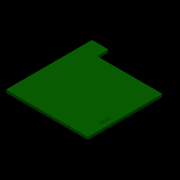
# Autodesk Inventor part: hw_DAA - PCB Power
Saved by Autodesk Inventor 2018 (Build 220112000, 112)
## iProperties
Created: 2024-03-13
Part Number: hw_DAA - PCB Power
Material: PCB
Document SubType Name: Modeling
Designer: cda1
Density: 4 g/cm^3
Appearance: PCB
Author: cda1
Autodesk Inventor part; units mm, degrees
ref_plane "YZ Plane" through (0, 0, 0) normal (1, 0, 0) x (0, 1, 0)
ref_plane "XZ Plane" through (0, 0, 0) normal (0, 1, 0) x (-1, 0, 0)
sketch "Boceto1" plane through (0, 0, 0) normal (0, 0, 1) x (1, 0, 0)
  line L0 (-26, 26) -> (26, 26)
  line L1 (26, 26) -> (26, -26)
  line L2 (26, -26) -> (-26, -26)
  line L3 (-26, -26) -> (-26, 26)
  line L4 (-26, 26) -> (26, -26) construction
  line L5 (26, 26) -> (-26, -26) construction
  point P0 (0, 0)
  dimension "d0" = 52
  dimension "d1" = 52
  constraints: 12 end point, 2 midpoint, 2 parallel, 1 horizontal, 1 perpendicular
  measures "d0" distance of L1.end L2.end
  measures "d1" distance of L0.end L1.end
extrude "Extrusión1" add sketch "Boceto1" against normal blind 1.742
fillet "Empalme1" radius 0.5 4 edges at (26, 26, -0.871) (-26, 26, -0.871) (-26, -26, -0.871) (26, -26, -0.871)
ref_plane "Plano de trabajo1" through (0, 0, -1.6) normal (0, 0, 1) x (1, 0, 0)
sketch "Boceto6" plane through (0, 0, 0) normal (0, 0, 1) x (1, 0, 0)
  line L0 (-25.5, 26) -> (25.5, 26) construction
  line L1 (-25.5, 26) -> (25.5, 26) construction
  line L2 (-15.5, 26) -> (26, 26)
  line L3 (26, 26) -> (26, 21.2)
  line L4 (26, 21.2) -> (-15.5, 21.2)
  line L5 (-15.5, 21.2) -> (-15.5, 26)
  line L6 (26, 25.5) -> (26, -25.5) projected
  point P0 (0, 0)
  dimension "d14" = 4.8
  dimension "d15" = 41.5
  constraints: 8 end point, 2 parallel, 2 point on line, 1 horizontal, 1 perpendicular
  measures "d14" distance of L4.end L2.start
  measures "d15" distance of L3.end L4.end
extrude "Extrusión4" cut sketch "Boceto6" against normal through all
sketch "Boceto7" plane through (0, 0, -1.742) normal (0, 0, -1) x (-1, 0, 0)
  line L0 (25.5, 26) -> (15.5, 26) projected
  arc A0 (26, 25.5) -> (25.5, 26) centre (25.5, 25.5) ccw projected
  line L1 (26, 25.5) -> (26, 28.5)
  line L2 (26, 28.5) -> (15.5, 28.5)
  line L3 (15.5, 28.5) -> (15.5, 26)
  point P0 (0, 0)
  dimension "d18" = 2.5
  constraints: 6 end point, 2 perpendicular, 1 vertical
  measures "d18" distance of L2.end L0.end
extrude "Extrusión5" add sketch "Boceto7" against normal up to surface (1.742 mm away)
sketch "Boceto9" plane through (0, 0, -1.742) normal (0, 0, -1) x (-1, 0, 0)
  circle A0 centre (-21.765, -9.26) radius 0.37 projected
  circle A1 centre (-23.035, -9.26) radius 0.37 projected
  circle A2 centre (-23.035, -10.53) radius 0.37 projected
  circle A3 centre (-21.765, -10.53) radius 0.37 projected
  circle A4 centre (-23.035, -11.8) radius 0.37 projected
  circle A5 centre (-21.765, -11.8) radius 0.37 projected
  circle A6 centre (-23.035, -13.07) radius 0.37 projected
  circle A7 centre (-21.765, -13.07) radius 0.37 projected
  circle A8 centre (-23.035, -14.34) radius 0.37 projected
  circle A9 centre (-21.765, -14.34) radius 0.37 projected
  point P0 (0, 0)
extrude "Extrusión6" cut sketch "Boceto9" against normal up to surface (1.742 mm away)
fillet "Empalme2" radius 0.5 4 edges at (26, 21.2, -0.871) (-15.5, 21.2, -0.871) (-15.5, 28.5, -0.871) (-26, 28.5, -0.871)
